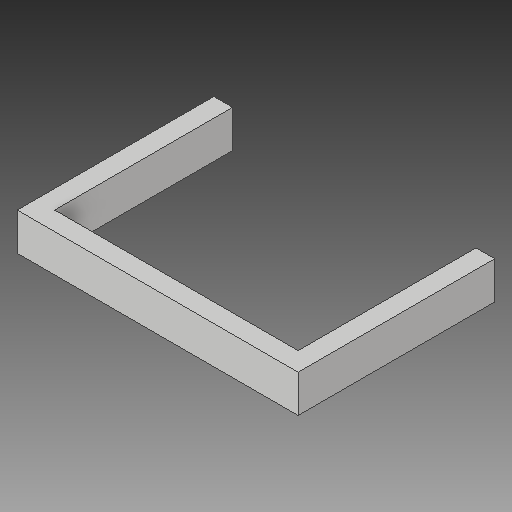
# Autodesk Inventor part: ShooterFrame
Saved by Autodesk Inventor 2017 SP1 (Build 210196100, 196)
## iProperties
Created: 2016-02-06
Part Number: ShooterFrame
Material: Generic
Document SubType Name: Modeling
Designer: steele
Density: 1 g/cm^3
Appearance: Default
Author: steele
Autodesk Inventor part; units mm, degrees
ref_plane "YZ Plane" through (0, 0, 0) normal (1, 0, 0) x (0, 1, 0)
ref_plane "XZ Plane" through (0, 0, 0) normal (0, 1, 0) x (-1, 0, 0)
sketch "Sketch1" plane through (0, 0, 0) normal (0, 1, 0) x (-1, 0, 0)
  line L0 (0, 0) -> (133.35, 0)
  line L1 (133.35, 0) -> (133.35, -190.5)
  line L2 (0, 0) -> (0, -190.5) construction
  line L3 (0, 0) -> (-133.35, 0)
  line L4 (-133.35, 0) -> (-133.35, -190.5)
  dimension "d0" = 133.35
  dimension "d1" = 190.5
  dimension "d2" = 190.5
  constraints: 10 end point, 2 symmetric about line, 1 horizontal, 1 perpendicular, 1 vertical
  measures "d0" distance of L0.start L0.end
  measures "d1" distance of L0.end L1.end
  measures "d2" distance of L0.start L2.end
ref_plane "Work Plane1" through (0, 0, -190.5) normal (0, 0, 1) x (1, 0, 0)
sketch "Sketch3" plane through (0, 0, -190.5) normal (0, 0, 1) x (1, 0, 0)
  line L0 (142.875, -19.05) -> (123.825, -19.05)
  line L1 (123.825, -19.05) -> (123.825, 19.05)
  line L2 (123.825, 19.05) -> (142.875, 19.05)
  line L3 (142.875, 19.05) -> (142.875, -19.05)
  line L4 (142.875, -19.05) -> (123.825, 19.05) construction
  line L5 (123.825, -19.05) -> (142.875, 19.05) construction
  line L6 (139.7, -15.875) -> (127, -15.875)
  line L7 (127, -15.875) -> (127, 15.875)
  line L8 (127, 15.875) -> (139.7, 15.875)
  line L9 (139.7, 15.875) -> (139.7, -15.875)
  line L10 (139.7, -15.875) -> (127, 15.875) construction
  line L11 (127, -15.875) -> (139.7, 15.875) construction
  point P0 (0, 0)
  point P1 (133.35, 0)
  dimension "d4" = 38.1
  dimension "d5" = 19.05
  dimension "d6" = 133.35
  dimension "d7" = 3.175
  dimension "d8" = 3.175
  constraints: 24 end point, 4 midpoint, 4 parallel, 2 horizontal, 2 perpendicular
  measures "d4" distance of L2.end L0.start
  measures "d5" distance of L0.start L0.end
  measures "d6" distance of point (133.35, 0) point (0, 0)
  measures "d7" distance between parallel lines of L2 L8
  measures "d8" distance between parallel lines of L3 L9
sweep "Sweep1" add profiles "Sketch3" path "Sketch1"
equation "\"d0\" = 0.5 * width"
equation "\"d1\" = length"
equation "\"d2\" = length"
equation "\"d4\" = tubingLength"
equation "\"d5\" = tubingWidth"
equation "\"d6\" = 0.5 * width"
equation "\"d7\" = tubeingWallWidth"
equation "\"d8\" = tubeingWallWidth"
equation "\"width\" = 266.7"
equation "\"length\" = 190.5"
equation "\"tubingWidth\" = 19.05"
equation "\"tubingLength\" = 38.1"
equation "\"tubeingWallWidth\" = 3.175"
equation "\"d3\" = -length"
body "Solid1"
